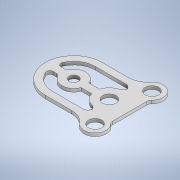
# Autodesk Inventor part: Part1
Saved by Autodesk Inventor 2021 (Build 250183000, 183)
## iProperties
Created: 2022-04-24
Part Number: Part1
Material: Generic
Document SubType Name: Modeling
Designer: hp
Density: 1 g/cm^3
Appearance: Default
Author: hp
Autodesk Inventor part; units mm, degrees
ref_plane "YZ Plane" through (0, 0, 0) normal (1, 0, 0) x (0, 1, 0)
ref_plane "XZ Plane" through (0, 0, 0) normal (0, 1, 0) x (-1, 0, 0)
ref_plane "XY Plane" through (0, 0, 0) normal (0, 0, 1) x (1, 0, 0)
sketch "Sketch1" plane through (0, 0, 0) normal (0, 1, 0) x (-1, 0, 0)
  arc A0 (176.3419, -210.5927) -> (175.3044, -30.5987) centre (175.3044, -120.5987) ccw
  line L0 (175.3044, -30.5987) -> (91.4725, -30.5987)
  line L1 (-2.1956, -66.2894) -> (-2.1956, -174.8751)
  line L2 (91.4505, -210.5927) -> (176.3419, -210.5927)
  arc A1 (44.9453, -8.483) -> (-6.6956, -55.5772) centre (17.8044, -30.5822) ccw
  arc A2 (-6.6956, -185.5872) -> (44.9372, -232.6914) centre (17.8044, -210.5822) ccw
  line L3 (265.3044, -138.5987) -> (263.4861, -138.5987)
  line L4 (263.4861, -102.5987) -> (265.3044, -102.5987)
  circle A3 centre (175.3044, -120.5987) radius 14.5
  line L5 (175.3044, -52.5987) -> (77.8044, -52.5987)
  line L6 (77.8044, -188.5987) -> (175.3044, -188.5987)
  arc A4 (237.9792, -94.2194) -> (175.3044, -52.5987) centre (175.3044, -120.5987) ccw
  arc A5 (175.3044, -188.5987) -> (237.9792, -146.978) centre (175.3044, -120.5987) ccw
  line L7 (228.7624, -133.0987) -> (217.1374, -133.0987)
  line L8 (217.1374, -108.0987) -> (228.7624, -108.0987)
  line L9 (139.9491, -108.0987) -> (106.0335, -108.0987)
  line L10 (106.0335, -133.0987) -> (139.9491, -133.0987)
  arc A6 (208.3305, -102.8356) -> (139.9491, -108.0987) centre (175.3044, -120.5987) ccw
  arc A7 (139.9491, -133.0987) -> (208.3305, -138.3619) centre (175.3044, -120.5987) ccw
  line L11 (62.8044, -67.5987) -> (62.8044, -62.504)
  line L12 (62.8044, -178.6935) -> (62.8044, -173.5987)
  arc A8 (106.0335, -108.0987) -> (74.0544, -77.0277) centre (62.8044, -120.5987) ccw
  arc A9 (74.0544, -164.1698) -> (106.0335, -133.0987) centre (62.8044, -120.5987) ccw
  circle A10 centre (62.8044, -120.5987) radius 21
  circle A11 centre (17.8044, -30.5822) radius 21
  circle A12 centre (17.8044, -210.5822) radius 21
  arc A13 (239.6919, -108.0987) -> (241.6431, -105.6593) centre (239.6919, -106.0987) ccw
  arc A14 (228.7624, -108.0987) -> (237.9792, -94.2194) centre (228.7624, -98.0987) ccw
  arc A15 (208.3305, -102.8356) -> (217.1374, -108.0987) centre (217.1374, -98.0987) ccw
  arc A16 (217.1374, -133.0987) -> (208.3305, -138.3619) centre (217.1374, -143.0987) ccw
  arc A17 (237.9792, -146.978) -> (228.7624, -133.0987) centre (228.7624, -143.0987) ccw
  arc A18 (77.8044, -52.5987) -> (62.8044, -67.5987) centre (77.8044, -67.5987) ccw
  arc A19 (62.8044, -173.5987) -> (77.8044, -188.5987) centre (77.8044, -173.5987) ccw
  arc A20 (62.8044, -62.504) -> (74.0544, -77.0277) centre (77.8044, -62.504) ccw
  arc A21 (74.0544, -164.1698) -> (62.8044, -178.6935) centre (77.8044, -178.6935) ccw
  arc A22 (44.9453, -8.483) -> (91.4725, -30.5987) centre (91.4725, 29.4013) ccw
  arc A23 (91.4505, -210.5927) -> (44.9372, -232.6914) centre (91.4505, -270.5927) ccw
  arc A24 (-2.1956, -66.2894) -> (-6.6956, -55.5772) centre (-17.1956, -66.2894) ccw
  arc A25 (-6.6956, -185.5872) -> (-2.1956, -174.8751) centre (-17.1956, -174.8751) ccw
  point P0 (0, 0)
  point P1 (-2.1956, -181.8594)
  point P2 (242.1457, -108.0987)
  point P3 (242.1457, -133.0987)
  point P4 (62.8044, -188.5987)
  point P5 (210.6598, -108.0987)
  point P6 (210.6598, -133.0987)
  point P7 (62.8044, -52.5987)
  point P8 (62.8044, -75.5987)
  point P9 (62.8044, -165.5987)
  point P10 (-2.1956, -59.3051)
  point P11 (52.8044, -30.5987)
  point P12 (52.8044, -210.5927)
  point P13 (63.0223, -65.0513)
  point P14 (63.0223, -176.1461)
  dimension "d0" = 180
  dimension "d1" = 20
  dimension "d2" = 20
  dimension "d3" = 42
  dimension "d4" = 70
  dimension "d5" = 42
  dimension "d6" = 70
  dimension "d7" = 112.5
  dimension "d8" = 90
  dimension "d9" = 90
  dimension "d10" = 25
  dimension "d11" = 90
  dimension "d12" = 68
  dimension "d13" = 77.5
  dimension "d14" = 37.5
  dimension "d15" = 37.5
  dimension "d16" = 29
  dimension "d17" = 45
  dimension "d18" = 45
  dimension "d19" = 42
  dimension "d20" = 25
  dimension "d21" = 77.5
  dimension "d22" = 112.5
  dimension "d23" = 112.5
  dimension "d24" = 45
  dimension "d25" = 68
  dimension "d26" = 2
  dimension "d27" = 10
  dimension "d28" = 15
  dimension "d29" = 60
  constraints: 57 point on circle, 26 centre point, 26 end point, 26 tangent, 15 point on line, 9 equal radius, 6 coincident, 3 horizontal, 3 parallel, 3 perpendicular
  measures "d0" distance of A2.centre A1.centre
  measures "d1" distance from line of L1 A1.centre
  measures "d2" distance from line of L1 A2.centre
  measures "d3" diameter of A11
  measures "d4" diameter of A1
  measures "d5" diameter of A12
  measures "d6" diameter of A2
  measures "d7" distance of A4.centre A8.centre
  measures "d8" distance from line of L0 A4.centre
  measures "d9" distance from line of L0 A8.centre
  measures "d10" distance between parallel lines of L7 L8
  measures "d11" radius of A0
  measures "d12" radius of A5
  measures "d13" distance between parallel lines of L0 L8
  measures "d14" radius of A7
  measures "d15" radius of A6
  measures "d16" diameter of A3
  measures "d17" radius of A9
  measures "d18" radius of A8
  measures "d19" diameter of A10
  measures "d20" distance between parallel lines of L10 L9
  measures "d21" distance between parallel lines of L0 L9
  measures "d22" distance of L5.start point (62.804, -52.599)
  measures "d23" distance of point (62.804, -188.599) L6.end
  measures "d24" horizontal distance of A8.centre A2.centre
  measures "d25" radius of A4
  measures "d26" radius of A13
  measures "d27" radius of A14
  measures "d28" radius of A18
  measures "d29" radius of A22
extrude "Extrusion1" add sketch "Sketch1" along normal blind 10
equation "\"d2\" = d1"
equation "\"d5\" = d3"
equation "\"d6\" = d4"
equation "\"d15\" = d14"
equation "\"d18\" = d17"
equation "\"d20\" = d10"
equation "\"d21\" = d13"
equation "\"d23\" = d22"
equation "\"d25\" = d12"
body "Solid1"
